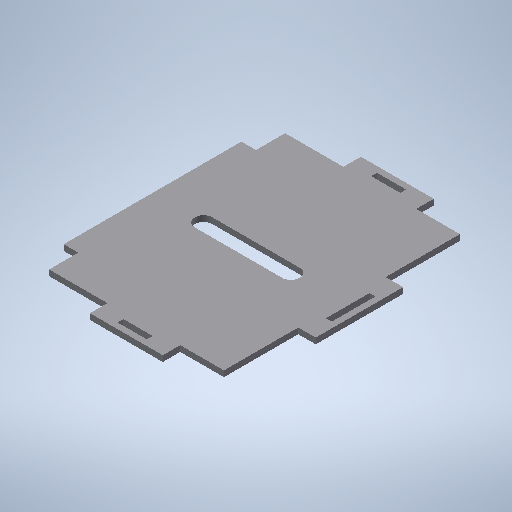
# Autodesk Inventor part: Parte intermedia
Saved by Autodesk Inventor 2025 (Build 290162000, 162)
## iProperties
Created: 2024-10-23
Part Number: Parte intermedia
Material: Generic
Document SubType Name: Modeling
Designer: feder
Density: 1 g/cm^3
Appearance: Default
Author: feder
Autodesk Inventor part; units mm, degrees
ref_plane "YZ Plane" through (0, 0, 0) normal (1, 0, 0) x (0, 1, 0)
ref_plane "XZ Plane" through (0, 0, 0) normal (0, 1, 0) x (-1, 0, 0)
ref_plane "XY Plane" through (0, 0, 0) normal (0, 0, 1) x (1, 0, 0)
sketch "Sketch1" plane through (0, 0, 0) normal (0, 1, 0) x (-1, 0, 0)
  line L0 (65, 81) -> (-65, 81)
  line L1 (-65, 81) -> (-65, -81)
  line L2 (-65, -81) -> (65, -81)
  line L3 (65, -81) -> (65, 81)
  point P0 (0, 0)
  point P1 (65, 0)
  point P2 (0, -81)
  dimension "d0" = 162
  dimension "d1" = 130
  constraints: 8 end point, 2 midpoint, 2 parallel, 1 horizontal, 1 horizontal alignment, 1 perpendicular, 1 vertical alignment
  measures "d0" distance of L2.end L0.start
  measures "d1" distance of L1.end L2.end
extrude "Extrusion1" add sketch "Sketch1" along normal blind 4
sketch "Sketch2" plane through (0, 4, 0) normal (0, 1, 0) x (1, 0, 0)
  circle A0 centre (-30, 0) radius 6
  circle A1 centre (30, 0) radius 6
  line L0 (-30, 6) -> (30, 6)
  line L1 (-30, -6) -> (30, -6)
  point P0 (0, 0)
  dimension "d4" = 12
  dimension "d5" = 12
  dimension "d6" = 30
  dimension "d7" = 30
  constraints: 4 end point, 4 point on circle, 2 centre point, 2 horizontal alignment, 1 horizontal, 1 parallel
  measures "d4" diameter of A0
  measures "d5" diameter of A1
  measures "d6" distance of point (0, 0) A0.centre
  measures "d7" distance of point (0, 0) A1.centre
extrude "Extrusion2" cut sketch "Sketch2" against normal through all
sketch "Sketch3" plane through (65, 0, 81) normal (1, 0, 0) x (0, 0, -1)
  line L0 (0, 4) -> (162, 4) projected
  line L1 (0, 0) -> (162, 0) projected
  line L2 (51, 4) -> (111, 4)
  line L3 (111, 4) -> (111, 0)
  line L4 (111, 0) -> (51, 0)
  line L5 (51, 0) -> (51, 4)
  point P0 (81, 0)
  point P1 (81, 0)
  dimension "d10" = 60
  dimension "d11" = 30
  constraints: 8 end point, 2 parallel, 2 point on line, 1 horizontal, 1 midpoint, 1 perpendicular
  measures "d10" distance between parallel lines of L5 L3
  measures "d11" distance from line of point (81, 0) L3
extrude "Extrusion3" add sketch "Sketch3" along normal blind 12
sketch "Sketch4" plane through (0, 4, 0) normal (0, 1, 0) x (1, 0, 0)
  line L0 (-65, -81) -> (65, -81) projected
  line L1 (-65, -81) -> (-55, -81)
  line L2 (-55, -81) -> (-55, -61)
  line L3 (-55, -61) -> (-65, -61)
  line L4 (-65, -61) -> (-65, -81)
  point P0 (0, 0)
  dimension "d14" = 20
  dimension "d15" = 10
  constraints: 8 end point, 2 parallel, 1 horizontal, 1 perpendicular
  measures "d14" distance of L1.end L2.end
  measures "d15" distance of L2.end L3.end
extrude "Extrusion4" cut sketch "Sketch4" against normal blind 4
mirror "Mirror1" about plane through (0, 0, 0) normal (0, 0, 1) of "Extrusion4"
sketch "Sketch5" plane through (65, 0, 81) normal (0, 0, 1) x (1, 0, 0)
  line L0 (-35, 4) -> (-95, 4) projected
  line L1 (-80, 4) -> (-30, 4)
  line L2 (-30, 4) -> (-30, 0)
  line L3 (-30, 0) -> (-80, 0)
  line L4 (-80, 0) -> (-80, 4)
  line L5 (0, 0) -> (0, 4) projected
  point P0 (-65, 0)
  point P1 (-30, 2)
  point P2 (-80, 2)
  point P3 (0, 2)
  point P4 (-55, 0)
  dimension "d18" = 50
  dimension "d19" = 55
  constraints: 8 end point, 4 midpoint, 2 parallel, 1 horizontal, 1 perpendicular, 1 point on line
  measures "d18" distance of point (-30, 2) point (-80, 2)
  measures "d19" horizontal distance of point (0, 2) point (-55, 0)
extrude "Extrusion5" add sketch "Sketch5" along normal blind 12
sketch "Sketch6" plane through (0, 4, 0) normal (0, 1, 0) x (1, 0, 0)
  line L0 (0, -85) -> (20, -85)
  line L1 (20, -85) -> (20, -89)
  line L2 (20, -89) -> (0, -89)
  line L3 (0, -89) -> (0, -85)
  line L4 (35, -81) -> (65, -81) projected
  line L5 (35, -81) -> (35, -93) projected
  point P0 (0, 0)
  point P1 (20, -87)
  dimension "d22" = 20
  dimension "d23" = 4
  dimension "d24" = 4
  dimension "d25" = 15
  constraints: 8 end point, 2 parallel, 1 horizontal, 1 midpoint, 1 perpendicular
  measures "d22" distance of L0.start L0.end
  measures "d23" distance of L0.end L1.end
  measures "d24" distance between parallel lines of L4 L0
  measures "d25" distance from line of L5 point (20, -87)
extrude "Extrusion6" cut sketch "Sketch6" against normal blind 12
mirror "Mirror2" about plane through (0, 0, 0) normal (0, 0, 1) of "Extrusion5", "Extrusion6"
sketch "Sketch7" plane through (0, 4, 0) normal (0, 1, 0) x (1, 0, 0)
  line L0 (69, 15) -> (73, 15)
  line L1 (73, 15) -> (73, -15)
  line L2 (73, -15) -> (69, -15)
  line L3 (69, -15) -> (69, 15)
  line L4 (65, 30) -> (65, 81) projected
  point P0 (0, 0)
  point P1 (69, 0)
  dimension "d28" = 4
  dimension "d29" = 4
  dimension "d30" = 30
  constraints: 8 end point, 2 parallel, 1 horizontal, 1 horizontal alignment, 1 midpoint, 1 perpendicular
  measures "d28" distance of L0.start L0.end
  measures "d29" distance from line of L4 L0.start
  measures "d30" distance of L0.end L1.end
extrude "Extrusion7" cut sketch "Sketch7" against normal blind 12
body "Solid1"
